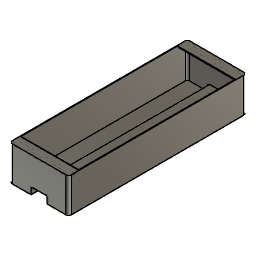
12Ga Tray v4 (Autodesk Fusion 360 design; units mm, degrees)
Autodesk Fusion 360 part; units mm, degrees
sketch "Sketch1" plane through (0, 0, 0) normal (0, 0, 1) x (1, 0, 0)
  line L0 (38.5, 128) -> (-38.5, 128)
  line L1 (-42.5, 124) -> (-42.5, -124)
  line L2 (-38.5, -128) -> (38.5, -128)
  line L3 (42.5, -124) -> (42.5, 124)
  line L4 (42.5, 128) -> (-42.5, -128) construction
  line L5 (-42.5, 128) -> (42.5, -128) construction
  arc A0 (-38.5, 128) -> (-42.5, 124) centre (-38.5, 124) ccw
  arc A1 (42.5, 124) -> (38.5, 128) centre (38.5, 124) ccw
  arc A2 (-42.5, -124) -> (-38.5, -128) centre (-38.5, -124) ccw
  arc A3 (38.5, -128) -> (42.5, -124) centre (38.5, -124) ccw
  dimension "d1" = 85
  dimension "d2" = 256
  dimension "d3" = 4
  dimension "d4" = 4
  dimension "d5" = 4
  dimension "d6" = 4
  constraint horizontal L0
  constraint perpendicular L0 L1
  constraint parallel L0 L2
  constraint parallel L1 L3
  constraint coincident L4 origin
  constraint coincident L5 origin
  constraint coincident L5.start L0
  constraint coincident L5.start L1
  constraint tangent L0 A0
  constraint tangent L1 A0
  constraint coincident L4.start L0
  constraint coincident L4.start L3
  constraint tangent L0 A1
  constraint tangent L3 A1
  constraint coincident L4.end L1
  constraint coincident L4.end L2
  constraint tangent L1 A2
  constraint tangent L2 A2
  constraint coincident L5.end L2
  constraint coincident L5.end L3
  constraint tangent L2 A3
  constraint tangent L3 A3
  measures "d1" distance of L4.end L5.end
  measures "d2" distance of L5.start L4.end
  measures "d3" radius of A0
  measures "d4" radius of A1
  measures "d5" radius of A2
  measures "d6" radius of A3
extrude "Extrude1" add sketch "Sketch1" along normal blind 50
sketch "Sketch4" plane through (0, -128, 0) normal (0, -1, 0) x (1, 0, 0)
  line L0 (-38.5, 0) -> (38.5, 0)
  line L1 (38.5, 0) -> (38.5, 50)
  line L2 (38.5, 50) -> (-38.5, 50)
  line L3 (-38.5, 50) -> (-38.5, 0)
  line L4 (-9.5, 10) -> (9.5, 10)
  line L5 (11.5, 8) -> (11.5, 0)
  line L6 (11.5, 0) -> (-11.5, 0)
  line L7 (-11.5, 0) -> (-11.5, 8)
  line L8 (42.5, 0) -> (42.5, 50)
  line L9 (-42.5, 0) -> (-42.5, 50)
  arc A0 (11.5, 8) -> (9.5, 10) centre (9.5, 8) ccw
  arc A1 (-9.5, 10) -> (-11.5, 8) centre (-9.5, 8) ccw
  dimension "d33" = 31
  dimension "d34" = 31
  dimension "d35" = 10
  dimension "d36" = 2
  constraint horizontal L4
  constraint vertical L5
  constraint horizontal L6
  constraint vertical L7
  constraint coincident L0 L5.end
  constraint tangent L5 A0
  constraint tangent L4 A0
  constraint tangent L7 A1
  constraint tangent L4 A1
  constraint equal A0 A1
  measures "d33" distance of L5 L8
  measures "d34" distance of L7 L9
  measures "d35" distance of L4 L6
  measures "d36" radius of A0
extrude "Extrude4" cut sketch "Sketch4" against normal blind 309 contours L0 L4 L5 L6 L7 A0 A1
sketch "Sketch5" plane through (0, 0, 50) normal (0, 0, 1) x (-1, 0, 0)
  arc A0 (-38.5, 128) -> (-42.5, 124) centre (-38.5, 124) ccw
  line L0 (-42.5, 124) -> (-42.5, -124)
  arc A1 (-42.5, -124) -> (-38.5, -128) centre (-38.5, -124) ccw
  line L1 (-38.5, -128) -> (38.5, -128)
  arc A2 (38.5, -128) -> (42.5, -124) centre (38.5, -124) ccw
  line L2 (42.5, -124) -> (42.5, 124)
  arc A3 (42.5, 124) -> (38.5, 128) centre (38.5, 124) ccw
  line L3 (38.5, 128) -> (-38.5, 128)
  line L4 (42.5, -113) -> (-42.5, -113)
  line L5 (42.5, 113) -> (-42.5, 113)
  dimension "d39" = 15
  dimension "d40" = 15
  constraint coincident L2 L4.start
  constraint coincident L0 L4.end
  constraint perpendicular L0 L4
  constraint coincident L2 L5.start
  constraint coincident L0 L5.end
  constraint perpendicular L0 L5
  measures "d39" distance of L1 L4
  measures "d40" distance of L3 L5
shell "Shell1" thickness 1 removed faces 1 at (-14.1667, 41.3333, 50)
extrude "Extrude5" add sketch "Sketch5" against normal blind 1.4 contours A0 L0 L2 A3 L3 L5 | L0 A1 L1 A2 L2 L4
sketch "Sketch6" plane through (-42.5, 0, 0) normal (-1, 0, 0) x (0, -1, 0)
  line L0 (-124, 50) -> (-124, 0)
  line L1 (-124, 0) -> (124, 0)
  line L2 (124, 0) -> (124, 50)
  line L3 (124, 50) -> (-124, 50)
  line L4 (113.5, 50) -> (112.5, 50)
  arc A0 (128.5, 34) -> (112.5, 50) centre (112.5, 34) ccw
  line L5 (0, 58.2501) -> (0, -6.7993) construction
  arc A1 (-112.5, 50) -> (-128.5, 34) centre (-112.5, 34) ccw
  dimension "d46" = 16
  constraint horizontal L4
  constraint coincident L3 L4.start
  constraint tangent L4 A0
  constraint perpendicular L1 L5
  constraint symmetric L4.end L5 A1.start
  constraint symmetric A0.start L5 A1.end
  constraint symmetric A0 L5 A1
  measures "d46" radius of A0
extrude "Extrude6" add sketch "Sketch6" against normal blind 85 contours L0 L3 A1 | L2 L3 L4 A0
named bodies: "12Ga Tray"
